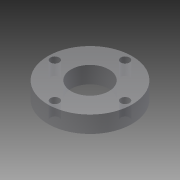
# Autodesk Inventor part: Spacer Plate 2
Saved by Autodesk Inventor 2013 (Build 170138000, 138)
## iProperties
Created: 2013-01-18
Part Number: Spacer Plate 2
Material: Polycarbonate, Clear
Document SubType Name: Modeling
Designer: actoennies
Mass: 36.4024 g
Surface Area: 95.0479 cm^2
Volume: 30.3353 cm^3
Density: 1.2 g/cm^3
Author: actoennies
Autodesk Inventor part; units mm, degrees
ref_plane "YZ Plane" through (0, 0, 0) normal (1, 0, 0) x (0, 1, 0)
ref_plane "XZ Plane" through (0, 0, 0) normal (0, 1, 0) x (-1, 0, 0)
ref_plane "XY Plane" through (0, 0, 0) normal (0, 0, 1) x (1, 0, 0)
sketch "Sketch1" plane through (0, 0, 0) normal (0, 1, 0) x (-1, 0, 0)
  circle A0 centre (0, 0) radius 14.2875
  circle A1 centre (0, 0) radius 26.543 construction
  circle A2 centre (0, 0) radius 31.75
  circle A3 centre (0, 26.543) radius 3.302
  circle A4 centre (26.543, 0) radius 3.302
  circle A5 centre (0, -26.543) radius 3.302
  circle A6 centre (-26.543, 0) radius 3.302
  dimension "d0" = 28.575
  dimension "d1" = 53.086
  dimension "d2" = 63.5
  dimension "d3" = 6.604
  dimension "d4" = 6.604
  dimension "d5" = 6.604
  dimension "d6" = 6.604
  constraints: 7 centre point, 4 point on circle, 3 coincident
  measures "d0" diameter of A0
  measures "d1" diameter of A1
  measures "d2" diameter of A2
  measures "d3" diameter of A3
  measures "d4" diameter of A4
  measures "d5" diameter of A5
  measures "d6" diameter of A6
extrude "Extrusion1" add sketch "Sketch1" along normal blind 12.7
body "Solid1"
